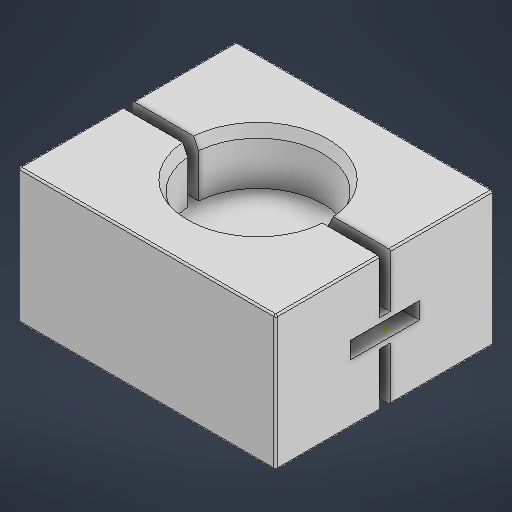
# Autodesk Inventor part: Base_Casing_A0645_v2
Saved by Autodesk Inventor 2026.2 (Build 302298010, 298A)
## iProperties
Created: 2025-09-05
Part Number: Base_Casing_A0645_v2
Material: Generic
Document SubType Name: Modeling
Designer: usman
Density: 1 g/cm^3
Appearance: Default
Author: usman
Autodesk Inventor part; units mm, degrees
ref_plane "YZ Plane" through (0, 0, 0) normal (1, 0, 0) x (0, 1, 0)
ref_plane "XZ Plane" through (0, 0, 0) normal (0, 1, 0) x (-1, 0, 0)
ref_plane "XY Plane" through (0, 0, 0) normal (0, 0, 1) x (1, 0, 0)
sketch "Sketch1" plane through (0, 0, 0) normal (1, 0, 0) x (0, 1, 0)
  line L0 (-39.75, 64.55) -> (39.75, 64.55)
  line L1 (39.75, 64.55) -> (39.75, -64.55)
  line L2 (39.75, -64.55) -> (-39.75, -64.55)
  line L3 (-39.75, -64.55) -> (-39.75, 64.55)
  line L4 (-39.75, 64.55) -> (39.75, -64.55) construction
  line L5 (39.75, 64.55) -> (-39.75, -64.55) construction
  point P0 (0, 0)
  dimension "d0" = 79.5
  dimension "d42" = 129.1
  constraints: 12 end point, 2 midpoint, 2 parallel, 1 horizontal, 1 perpendicular
  measures "d0" distance of L1.end L2.end
  measures "d42" distance of L2.end L0.start
extrude "Extrusion1" add sketch "Sketch1" along normal blind 152.4
sketch "Sketch2" plane through (152.4, 0, 0) normal (1, 0, 0) x (0, 0, -1)
  line L0 (-20.5, -5) -> (20.5, -5)
  line L1 (20.5, -5) -> (20.5, 5)
  line L2 (20.5, 5) -> (-20.5, 5)
  line L3 (-20.5, 5) -> (-20.5, -5)
  line L4 (-20.5, -5) -> (20.5, 5) construction
  line L5 (20.5, -5) -> (-20.5, 5) construction
  point P0 (0, 0)
  dimension "d4" = 10
  dimension "d5" = 41
  constraints: 12 end point, 2 midpoint, 2 parallel, 1 horizontal, 1 perpendicular
  measures "d4" distance of L0.end L1.end
  measures "d5" distance of L1.end L2.end
extrude "Extrusion2" cut sketch "Sketch2" against normal through all
sketch "Sketch3" plane through (152.4, 0, 0) normal (1, 0, 0) x (0, 0, -1)
  point P0 (0, 0)
sketch "Sketch4" plane through (0, 39.75, 64.55) normal (0, 1, 0) x (1, 0, 0)
  line L0 (115.0902, 28.6551) -> (39.7066, 100.4449) construction
  line L1 (39.7066, 28.6551) -> (115.0902, 100.4449) construction
  line L2 (0, 129.1) -> (0, 0) projected
  line L3 (0, 129.1) -> (152.4, 129.1) projected
  circle A0 centre (77.3984, 64.55) radius 38.5
  line L4 (152.4, 129.1) -> (152.4, 0) projected
  point P0 (0, 64.55)
  dimension "d23" = 77
  dimension "d24" = 129.1
  dimension "d25" = 64.55
  dimension "d43" = 77.3984
  dimension "d44" = 75.0016
  constraints: 4 end point, 2 midpoint, 1 centre point, 1 coincident
  measures "d23" diameter of A0
  measures "d24" distance of L2.start L2.end
  measures "d25" vertical distance of point (77.398, 64.55) L2.end
  measures "d43" distance from line of L2 point (77.398, 64.55)
  measures "d44" distance from line of L4 point (77.398, 64.55)
extrude "Extrusion3" cut sketch "Sketch4" against normal blind 31.7
mirror "Mirror1" about plane through (0, 0, 0) normal (0, 1, 0) of "Extrusion3"
sketch "Sketch5" plane through (0, 0, 0) normal (-1, 0, 0) x (0, 0, 1)
  line L0 (-64.55, 39.75) -> (64.55, 39.75) projected
  line L1 (-3.25, 8.05) -> (3.25, 8.05)
  line L2 (3.25, 8.05) -> (3.25, 39.75)
  line L3 (3.25, 39.75) -> (-3.25, 39.75)
  line L4 (-3.25, 39.75) -> (-3.25, 8.05)
  line L5 (-3.25, 8.05) -> (3.25, 39.75) construction
  line L6 (3.25, 8.05) -> (-3.25, 39.75) construction
  point P0 (0, 0)
  point P1 (0, 23.9)
  point P2 (-3.25, 39.75)
  dimension "d12" = 3.25
  dimension "d13" = 31.7
  constraints: 12 end point, 2 midpoint, 2 parallel, 1 horizontal, 1 perpendicular, 1 point on line
  measures "d12" distance from line of point (0, 23.9) L2
  measures "d13" distance of L1.end L2.end
extrude "Extrusion4" cut sketch "Sketch5" against normal through all
mirror "Mirror2" about plane through (0, 0, 0) normal (0, 1, 0) of "Extrusion4"
sketch "Sketch6" plane through (0, 0, 0) normal (-1, 0, 0) x (0, 0, 1)
  line L0 (-53.6471, 38.1768) -> (-14.1529, 38.1768) construction
  line L1 (-14.1529, 38.1768) -> (-14.1529, 7.4202) construction
  line L2 (-14.1529, 7.4202) -> (-53.6471, 7.4202) construction
  line L3 (-53.6471, 7.4202) -> (-53.6471, 38.1768) construction
  line L4 (-64.55, 39.75) -> (-3.25, 39.75) projected
  line L5 (-43.049, 25.8134) -> (-43.049, 31.9094)
  line L6 (-43.049, 31.9094) -> (-42.0942, 31.9094)
  spline S0 degree 2 poles (-42.0942, 31.9094) (-41.2599, 31.9094) (-40.873, 31.8039) knots 0 0 0 1 1 1
  spline S1 degree 2 poles (-40.873, 31.8039) (-40.3302, 31.6581) (-39.6819, 30.8691) (-39.6819, 30.3364) knots 0 0 0 1 2 2 2
  spline S2 degree 2 poles (-39.6819, 30.3364) (-39.6819, 29.9846) (-39.9734, 29.4167) (-40.3051, 29.1705) knots 0 0 0 1 2 2 2
  spline S3 degree 2 poles (-40.3051, 29.1705) (-39.7472, 28.9091) (-39.2346, 28.1252) (-39.2346, 27.5924) knots 0 0 0 1 2 2 2
  spline S4 degree 2 poles (-39.2346, 27.5924) (-39.2346, 27.0748) (-39.7673, 26.2305) (-40.6016, 25.8134) (-41.3403, 25.8134) knots 0 0 0 1 2 3 3 3
  line L7 (-41.3403, 25.8134) -> (-43.049, 25.8134)
  line L8 (-41.8881, 28.482) -> (-41.8881, 26.919)
  line L9 (-41.8881, 26.919) -> (-41.5966, 26.919)
  spline S5 degree 2 poles (-41.5966, 26.919) (-40.878, 26.919) (-40.3754, 27.2859) (-40.3754, 27.6327) knots 0 0 0 1 2 2 2
  spline S6 degree 2 poles (-40.3754, 27.6327) (-40.3754, 28.0246) (-40.9634, 28.482) (-41.6469, 28.482) knots 0 0 0 1 2 2 2
  line L10 (-41.6469, 28.482) -> (-41.8881, 28.482)
  line L11 (-41.8881, 30.8038) -> (-41.8881, 29.5172)
  line L12 (-41.8881, 29.5172) -> (-41.6368, 29.5172)
  spline S7 degree 2 poles (-41.6368, 29.5172) (-41.2147, 29.5172) (-40.8026, 29.8741) (-40.8026, 30.1806) knots 0 0 0 1 2 2 2
  spline S8 degree 2 poles (-40.8026, 30.1806) (-40.8026, 30.4671) (-41.1896, 30.8038) (-41.5916, 30.8038) knots 0 0 0 1 2 2 2
  line L13 (-41.5916, 30.8038) -> (-41.8881, 30.8038)
  line L14 (-34.9227, 30.3213) -> (-33.792, 30.3213)
  line L15 (-33.792, 30.3213) -> (-33.792, 25.8134)
  line L16 (-33.792, 25.8134) -> (-34.9227, 25.8134)
  line L17 (-34.9227, 25.8134) -> (-34.9227, 26.2908)
  spline S9 degree 2 poles (-34.9227, 26.2908) (-35.2544, 25.9742) (-35.9178, 25.6978) (-36.3098, 25.6978) knots 0 0 0 1 2 2 2
  spline S10 degree 2 poles (-36.3098, 25.6978) (-37.1792, 25.6978) (-38.4557, 27.0547) (-38.4557, 28.0598) knots 0 0 0 1 2 2 2
  spline S11 degree 2 poles (-38.4557, 28.0598) (-38.4557, 29.1051) (-37.2244, 30.4369) (-36.3399, 30.4369) knots 0 0 0 1 2 2 2
  spline S12 degree 2 poles (-36.3399, 30.4369) (-35.9379, 30.4369) (-35.2242, 30.1304) (-34.9227, 29.8238) knots 0 0 0 1 2 2 2
  line L18 (-34.9227, 29.8238) -> (-34.9227, 30.3213)
  spline S13 degree 2 poles (-36.1138, 29.3916) (-36.6364, 29.3916) (-37.3299, 28.6528) (-37.3299, 28.0699) knots 0 0 0 1 2 2 2
  spline S14 degree 2 poles (-37.3299, 28.0699) (-37.3299, 27.4869) (-36.6213, 26.7331) (-36.1087, 26.7331) knots 0 0 0 1 2 2 2
  spline S15 degree 2 poles (-36.1087, 26.7331) (-35.576, 26.7331) (-34.8724, 27.4769) (-34.8724, 28.0749) knots 0 0 0 1 2 2 2
  spline S16 degree 2 poles (-34.8724, 28.0749) (-34.8724, 28.6629) (-35.576, 29.3916) (-36.1138, 29.3916) knots 0 0 0 1 2 2 2
  line L19 (-29.8921, 29.6881) -> (-30.5907, 28.9896)
  spline S17 degree 2 poles (-30.5907, 28.9896) (-31.0128, 29.4117) (-31.3596, 29.4117) knots 0 0 0 1 1 1
  spline S18 degree 2 poles (-31.3596, 29.4117) (-31.5506, 29.4117) (-31.7667, 29.2509) (-31.7667, 29.1303) knots 0 0 0 1 2 2 2
  spline S19 degree 2 poles (-31.7667, 29.1303) (-31.7667, 29.0398) (-31.631, 28.884) (-31.3596, 28.7534) knots 0 0 0 1 2 2 2
  line L20 (-31.3596, 28.7534) -> (-30.9475, 28.5473)
  spline S20 degree 2 poles (-30.9475, 28.5473) (-30.2942, 28.2257) (-29.8067, 27.5522) (-29.8067, 27.0999) knots 0 0 0 1 2 2 2
  spline S21 degree 2 poles (-29.8067, 27.0999) (-29.8067, 26.5019) (-30.6862, 25.6978) (-31.4299, 25.6978) knots 0 0 0 1 2 2 2
  spline S22 degree 2 poles (-31.4299, 25.6978) (-32.4149, 25.6978) (-33.0029, 26.4667) knots 0 0 0 1 1 1
  line L21 (-33.0029, 26.4667) -> (-32.3094, 27.2256)
  spline S23 degree 2 poles (-32.3094, 27.2256) (-32.1084, 26.9944) (-31.5757, 26.708) (-31.3696, 26.708) knots 0 0 0 1 2 2 2
  spline S24 degree 2 poles (-31.3696, 26.708) (-31.1435, 26.708) (-30.8721, 26.924) (-30.8721, 27.0648) knots 0 0 0 1 2 2 2
  spline S25 degree 2 poles (-30.8721, 27.0648) (-30.8721, 27.3261) (-31.3646, 27.5723) knots 0 0 0 1 1 1
  line L22 (-31.3646, 27.5723) -> (-31.7465, 27.7633)
  spline S26 degree 2 poles (-31.7465, 27.7633) (-32.8371, 28.3161) (-32.8371, 29.1453) knots 0 0 0 1 1 1
  spline S27 degree 2 poles (-32.8371, 29.1453) (-32.8371, 29.6781) (-32.0129, 30.4369) (-31.3747, 30.4369) knots 0 0 0 1 2 2 2
  spline S28 degree 2 poles (-31.3747, 30.4369) (-30.9324, 30.4369) (-30.1585, 30.0499) (-29.8921, 29.6881) knots 0 0 0 1 2 2 2
  line L23 (-24.3992, 27.7432) -> (-28.0276, 27.7432)
  spline S29 degree 2 poles (-28.0276, 27.7432) (-27.9472, 27.2608) (-27.2638, 26.6929) (-26.7361, 26.6929) knots 0 0 0 1 2 2 2
  spline S30 degree 2 poles (-26.7361, 26.6929) (-26.1028, 26.6929) (-25.6455, 27.1351) knots 0 0 0 1 1 1
  line L24 (-25.6455, 27.1351) -> (-24.6957, 26.6878)
  spline S31 degree 2 poles (-24.6957, 26.6878) (-25.0525, 26.1853) (-26.0476, 25.6978) (-26.731, 25.6978) knots 0 0 0 1 2 2 2
  spline S32 degree 2 poles (-26.731, 25.6978) (-27.7914, 25.6978) (-29.1232, 27.0346) (-29.1232, 28.0447) knots 0 0 0 1 2 2 2
  spline S33 degree 2 poles (-29.1232, 28.0447) (-29.1232, 29.075) (-27.7914, 30.4369) (-26.7914, 30.4369) knots 0 0 0 1 2 2 2
  spline S34 degree 2 poles (-26.7914, 30.4369) (-25.7259, 30.4369) (-24.3942, 29.075) (-24.3942, 27.9593) knots 0 0 0 1 2 2 2
  line L25 (-24.3942, 27.9593) -> (-24.3992, 27.7432)
  spline S35 degree 2 poles (-25.5299, 28.6327) (-25.6405, 29.0097) (-26.2988, 29.477) (-26.7361, 29.477) knots 0 0 0 1 2 2 2
  spline S36 degree 2 poles (-26.7361, 29.477) (-27.2085, 29.477) (-27.5653, 29.2157) knots 0 0 0 1 1 1
  spline S37 degree 2 poles (-27.5653, 29.2157) (-27.7864, 29.0499) (-27.9774, 28.6327) knots 0 0 0 1 1 1
  line L26 (-27.9774, 28.6327) -> (-25.5299, 28.6327)
  line L27 (-48.5721, 21.5476) -> (-47.4464, 21.5476)
  line L28 (-47.4464, 21.5476) -> (-46.0292, 17.296)
  line L29 (-46.0292, 17.296) -> (-44.6019, 21.5476)
  line L30 (-44.6019, 21.5476) -> (-43.4762, 21.5476)
  line L31 (-43.4762, 21.5476) -> (-42.456, 15.4516)
  line L32 (-42.456, 15.4516) -> (-43.5767, 15.4516)
  line L33 (-43.5767, 15.4516) -> (-44.225, 19.3012)
  line L34 (-44.225, 19.3012) -> (-45.5216, 15.4516)
  line L35 (-45.5216, 15.4516) -> (-46.5468, 15.4516)
  line L36 (-46.5468, 15.4516) -> (-47.8283, 19.3012)
  line L37 (-47.8283, 19.3012) -> (-48.4967, 15.4516)
  line L38 (-48.4967, 15.4516) -> (-49.6275, 15.4516)
  line L39 (-49.6275, 15.4516) -> (-48.5721, 21.5476)
  line L40 (-38.32, 19.9595) -> (-37.1892, 19.9595)
  line L41 (-37.1892, 19.9595) -> (-37.1892, 15.4516)
  line L42 (-37.1892, 15.4516) -> (-38.32, 15.4516)
  line L43 (-38.32, 15.4516) -> (-38.32, 15.929)
  spline S38 degree 2 poles (-38.32, 15.929) (-38.6517, 15.6124) (-39.315, 15.336) (-39.707, 15.336) knots 0 0 0 1 2 2 2
  spline S39 degree 2 poles (-39.707, 15.336) (-40.5765, 15.336) (-41.8529, 16.6929) (-41.8529, 17.698) knots 0 0 0 1 2 2 2
  spline S40 degree 2 poles (-41.8529, 17.698) (-41.8529, 18.7433) (-40.6217, 20.0751) (-39.7372, 20.0751) knots 0 0 0 1 2 2 2
  spline S41 degree 2 poles (-39.7372, 20.0751) (-39.3351, 20.0751) (-38.6215, 19.7685) (-38.32, 19.462) knots 0 0 0 1 2 2 2
  line L44 (-38.32, 19.462) -> (-38.32, 19.9595)
  spline S42 degree 2 poles (-39.511, 19.0298) (-40.0337, 19.0298) (-40.7272, 18.291) (-40.7272, 17.7081) knots 0 0 0 1 2 2 2
  spline S43 degree 2 poles (-40.7272, 17.7081) (-40.7272, 17.1251) (-40.0186, 16.3713) (-39.506, 16.3713) knots 0 0 0 1 2 2 2
  spline S44 degree 2 poles (-39.506, 16.3713) (-38.9733, 16.3713) (-38.2697, 17.115) (-38.2697, 17.7131) knots 0 0 0 1 2 2 2
  spline S45 degree 2 poles (-38.2697, 17.7131) (-38.2697, 18.3011) (-38.9733, 19.0298) (-39.511, 19.0298) knots 0 0 0 1 2 2 2
  line L45 (-32.7165, 19.9595) -> (-31.5857, 19.9595)
  line L46 (-31.5857, 19.9595) -> (-31.5857, 16.0999)
  spline S46 degree 2 poles (-31.5857, 16.0999) (-31.5857, 14.9541) (-32.0481, 14.4163) knots 0 0 0 1 1 1
  spline S47 degree 2 poles (-32.0481, 14.4163) (-32.6612, 13.6876) (-33.9075, 13.6876) knots 0 0 0 1 1 1
  spline S48 degree 2 poles (-33.9075, 13.6876) (-34.5709, 13.6876) (-35.4705, 14.0193) (-36.0937, 14.6626) (-36.2444, 15.1199) knots 0 0 0 1 2 3 3 3
  line L47 (-36.2444, 15.1199) -> (-34.9981, 15.1199)
  spline S49 degree 2 poles (-34.9981, 15.1199) (-34.8322, 14.9289) (-34.3096, 14.738) (-33.9528, 14.738) knots 0 0 0 1 2 2 2
  spline S50 degree 2 poles (-33.9528, 14.738) (-33.5005, 14.738) (-32.9426, 15.0194) (-32.7165, 15.4667) (-32.7165, 16.0145) knots 0 0 0 1 2 3 3 3
  spline S51 degree 2 poles (-32.7165, 16.0145) (-33.013, 15.7129) (-33.6663, 15.4516) (-34.0834, 15.4516) knots 0 0 0 1 2 2 2
  spline S52 degree 2 poles (-34.0834, 15.4516) (-34.988, 15.4516) (-36.2394, 16.7633) (-36.2394, 17.7633) knots 0 0 0 1 2 2 2
  spline S53 degree 2 poles (-36.2394, 17.7633) (-36.2394, 18.8388) (-35.576, 19.4871) knots 0 0 0 1 1 1
  spline S54 degree 2 poles (-35.576, 19.4871) (-34.978, 20.0751) (-34.1437, 20.0751) knots 0 0 0 1 1 1
  spline S55 degree 2 poles (-34.1437, 20.0751) (-33.7568, 20.0751) (-33.0632, 19.7886) (-32.7165, 19.462) knots 0 0 0 1 2 2 2
  line L48 (-32.7165, 19.462) -> (-32.7165, 19.9595)
  spline S56 degree 2 poles (-33.8824, 19.0197) (-34.4201, 19.0197) (-35.1137, 18.3011) (-35.1137, 17.7583) knots 0 0 0 1 2 2 2
  spline S57 degree 2 poles (-35.1137, 17.7583) (-35.1137, 17.1955) (-34.4, 16.4768) (-33.8623, 16.4768) knots 0 0 0 1 2 2 2
  spline S58 degree 2 poles (-33.8623, 16.4768) (-33.3396, 16.4768) (-32.6562, 17.1804) (-32.6562, 17.7533) knots 0 0 0 1 2 2 2
  spline S59 degree 2 poles (-32.6562, 17.7533) (-32.6562, 18.3162) (-33.3447, 19.0197) (-33.8824, 19.0197) knots 0 0 0 1 2 2 2
  line L49 (-30.4399, 19.9595) -> (-29.3092, 19.9595)
  line L50 (-29.3092, 19.9595) -> (-29.3092, 19.4972)
  spline S60 degree 2 poles (-29.3092, 19.4972) (-28.9222, 19.8238) (-28.299, 20.0751) (-27.9724, 20.0751) knots 0 0 0 1 2 2 2
  spline S61 degree 2 poles (-27.9724, 20.0751) (-27.2989, 20.0751) (-26.8316, 19.6077) knots 0 0 0 1 1 1
  spline S62 degree 2 poles (-26.8316, 19.6077) (-26.4396, 19.2107) (-26.4396, 18.4317) knots 0 0 0 1 1 1
  line L51 (-26.4396, 18.4317) -> (-26.4396, 15.4516)
  line L52 (-26.4396, 15.4516) -> (-27.5603, 15.4516)
  line L53 (-27.5603, 15.4516) -> (-27.5603, 17.4266)
  spline S63 degree 2 poles (-27.5603, 17.4266) (-27.5603, 18.2307) (-27.706, 18.7634) (-28.0628, 19.0398) (-28.3292, 19.0398) knots 0 0 0 1 2 3 3 3
  spline S64 degree 2 poles (-28.3292, 19.0398) (-28.6709, 19.0398) (-29.1634, 18.5825) (-29.2589, 18.1754) knots 0 0 0 1 2 2 2
  spline S65 degree 2 poles (-29.2589, 18.1754) (-29.3092, 17.9644) (-29.3092, 17.2608) knots 0 0 0 1 1 1
  line L54 (-29.3092, 17.2608) -> (-29.3092, 15.4516)
  line L55 (-29.3092, 15.4516) -> (-30.4399, 15.4516)
  line L56 (-30.4399, 15.4516) -> (-30.4399, 19.9595)
  line L57 (-20.831, 17.3814) -> (-24.4595, 17.3814)
  spline S66 degree 2 poles (-24.4595, 17.3814) (-24.3791, 16.8989) (-23.6956, 16.3311) (-23.1679, 16.3311) knots 0 0 0 1 2 2 2
  spline S67 degree 2 poles (-23.1679, 16.3311) (-22.5347, 16.3311) (-22.0774, 16.7733) knots 0 0 0 1 1 1
  line L58 (-22.0774, 16.7733) -> (-21.1275, 16.326)
  spline S68 degree 2 poles (-21.1275, 16.326) (-21.4844, 15.8235) (-22.4794, 15.336) (-23.1629, 15.336) knots 0 0 0 1 2 2 2
  spline S69 degree 2 poles (-23.1629, 15.336) (-24.2233, 15.336) (-25.5551, 16.6728) (-25.5551, 17.6829) knots 0 0 0 1 2 2 2
  spline S70 degree 2 poles (-25.5551, 17.6829) (-25.5551, 18.7132) (-24.2233, 20.0751) (-23.2232, 20.0751) knots 0 0 0 1 2 2 2
  spline S71 degree 2 poles (-23.2232, 20.0751) (-22.1578, 20.0751) (-20.826, 18.7132) (-20.826, 17.5975) knots 0 0 0 1 2 2 2
  line L59 (-20.826, 17.5975) -> (-20.831, 17.3814)
  spline S72 degree 2 poles (-21.9618, 18.2709) (-22.0724, 18.6478) (-22.7307, 19.1152) (-23.1679, 19.1152) knots 0 0 0 1 2 2 2
  spline S73 degree 2 poles (-23.1679, 19.1152) (-23.6403, 19.1152) (-23.9971, 18.8539) knots 0 0 0 1 1 1
  spline S74 degree 2 poles (-23.9971, 18.8539) (-24.2183, 18.688) (-24.4092, 18.2709) knots 0 0 0 1 1 1
  line L60 (-24.4092, 18.2709) -> (-21.9618, 18.2709)
  line L61 (-19.7757, 21.623) -> (-18.6449, 21.623)
  line L62 (-18.6449, 21.623) -> (-18.6449, 19.9595)
  line L63 (-18.6449, 19.9595) -> (-17.9715, 19.9595)
  line L64 (-17.9715, 19.9595) -> (-17.9715, 18.9846)
  line L65 (-17.9715, 18.9846) -> (-18.6449, 18.9846)
  line L66 (-18.6449, 18.9846) -> (-18.6449, 15.4516)
  line L67 (-18.6449, 15.4516) -> (-19.7757, 15.4516)
  line L68 (-19.7757, 15.4516) -> (-19.7757, 18.9846)
  line L69 (-19.7757, 18.9846) -> (-20.3536, 18.9846)
  line L70 (-20.3536, 18.9846) -> (-20.3536, 19.9595)
  line L71 (-20.3536, 19.9595) -> (-19.7757, 19.9595)
  line L72 (-19.7757, 19.9595) -> (-19.7757, 21.623)
  point P0 (0, 0)
  point P1 (-33.9, 39.75)
  point P2 (-33.9, 38.1768)
  dimension "d0" = 79.5
  dimension "d42" = 129.1
  dimension "d26" = 0
  constraints: 2 midpoint, 2 other
  measures "d26" horizontal distance of point (-33.9, 39.75) point (-33.9, 38.177)
sketch "Sketch7" plane through (0, 0, 0) normal (-1, 0, 0) x (0, 0, 1)
  line L0 (15.2014, 37.9215) -> (52.5986, 37.9215) construction
  line L1 (52.5986, 37.9215) -> (52.5986, 6.8154) construction
  line L2 (52.5986, 6.8154) -> (15.2014, 6.8154) construction
  line L3 (15.2014, 6.8154) -> (15.2014, 37.9215) construction
  line L4 (-52.3897, -8.5629) -> (-15.4103, -8.5629) construction
  line L5 (-15.4103, -8.5629) -> (-15.4103, -37.9215) construction
  line L6 (-15.4103, -37.9215) -> (-52.3897, -37.9215) construction
  line L7 (-52.3897, -37.9215) -> (-52.3897, -8.5629) construction
  line L8 (3.25, 39.75) -> (64.55, 39.75) projected
  line L9 (-3.25, -39.75) -> (-64.55, -39.75) projected
  line L10 (25.8516, 25.0873) -> (25.0425, 24.3133)
  spline S0 degree 2 poles (25.0425, 24.3133) (24.2132, 25.1878) (23.178, 25.1878) knots 0 0 0 1 1 1
  spline S1 degree 2 poles (23.178, 25.1878) (22.3035, 25.1878) (21.1074, 23.9967) (21.1074, 23.1223) knots 0 0 0 1 2 2 2
  spline S2 degree 2 poles (21.1074, 23.1223) (21.1074, 22.5142) (21.6351, 21.5694) (22.6051, 21.0316) (23.1981, 21.0316) knots 0 0 0 1 2 3 3 3
  spline S3 degree 2 poles (23.1981, 21.0316) (23.7006, 21.0316) (24.5399, 21.4085) (25.0425, 21.9061) knots 0 0 0 1 2 2 2
  line L11 (25.0425, 21.9061) -> (25.8264, 21.0869)
  spline S4 degree 2 poles (25.8264, 21.0869) (25.153, 20.4235) (23.9519, 19.916) (23.178, 19.916) knots 0 0 0 1 2 2 2
  spline S5 degree 2 poles (23.178, 19.916) (21.7557, 19.916) (19.9465, 21.7151) (19.9465, 23.1273) knots 0 0 0 1 2 2 2
  spline S6 degree 2 poles (19.9465, 23.1273) (19.9465, 24.0369) (20.7707, 25.4541) (22.3086, 26.3135) (23.1931, 26.3135) knots 0 0 0 1 2 3 3 3
  spline S7 degree 2 poles (23.1931, 26.3135) (23.9519, 26.3135) (25.344, 25.6752) (25.8516, 25.0873) knots 0 0 0 1 2 2 2
  line L12 (30.073, 24.5746) -> (31.2038, 24.5746)
  line L13 (31.2038, 24.5746) -> (31.2038, 20.0667)
  line L14 (31.2038, 20.0667) -> (30.073, 20.0667)
  line L15 (30.073, 20.0667) -> (30.073, 20.5442)
  spline S8 degree 2 poles (30.073, 20.5442) (29.7414, 20.2275) (29.078, 19.9511) (28.686, 19.9511) knots 0 0 0 1 2 2 2
  spline S9 degree 2 poles (28.686, 19.9511) (27.8166, 19.9511) (26.5401, 21.308) (26.5401, 22.3131) knots 0 0 0 1 2 2 2
  spline S10 degree 2 poles (26.5401, 22.3131) (26.5401, 23.3585) (27.7713, 24.6902) (28.6558, 24.6902) knots 0 0 0 1 2 2 2
  spline S11 degree 2 poles (28.6558, 24.6902) (29.0579, 24.6902) (29.7715, 24.3837) (30.073, 24.0771) knots 0 0 0 1 2 2 2
  line L16 (30.073, 24.0771) -> (30.073, 24.5746)
  spline S12 degree 2 poles (28.882, 23.6449) (28.3593, 23.6449) (27.6658, 22.9062) (27.6658, 22.3232) knots 0 0 0 1 2 2 2
  spline S13 degree 2 poles (27.6658, 22.3232) (27.6658, 21.7402) (28.3744, 20.9864) (28.887, 20.9864) knots 0 0 0 1 2 2 2
  spline S14 degree 2 poles (28.887, 20.9864) (29.4197, 20.9864) (30.1233, 21.7302) (30.1233, 22.3282) knots 0 0 0 1 2 2 2
  spline S15 degree 2 poles (30.1233, 22.3282) (30.1233, 22.9162) (29.4197, 23.6449) (28.882, 23.6449) knots 0 0 0 1 2 2 2
  line L17 (35.1036, 23.9414) -> (34.4051, 23.2429)
  spline S16 degree 2 poles (34.4051, 23.2429) (33.9829, 23.665) (33.6362, 23.665) knots 0 0 0 1 1 1
  spline S17 degree 2 poles (33.6362, 23.665) (33.4452, 23.665) (33.2291, 23.5042) (33.2291, 23.3836) knots 0 0 0 1 2 2 2
  spline S18 degree 2 poles (33.2291, 23.3836) (33.2291, 23.2931) (33.3648, 23.1373) (33.6362, 23.0067) knots 0 0 0 1 2 2 2
  line L18 (33.6362, 23.0067) -> (34.0483, 22.8006)
  spline S19 degree 2 poles (34.0483, 22.8006) (34.7016, 22.479) (35.1891, 21.8056) (35.1891, 21.3533) knots 0 0 0 1 2 2 2
  spline S20 degree 2 poles (35.1891, 21.3533) (35.1891, 20.7552) (34.3096, 19.9511) (33.5658, 19.9511) knots 0 0 0 1 2 2 2
  spline S21 degree 2 poles (33.5658, 19.9511) (32.5808, 19.9511) (31.9928, 20.72) knots 0 0 0 1 1 1
  line L19 (31.9928, 20.72) -> (32.6863, 21.4789)
  spline S22 degree 2 poles (32.6863, 21.4789) (32.8874, 21.2477) (33.4201, 20.9613) (33.6261, 20.9613) knots 0 0 0 1 2 2 2
  spline S23 degree 2 poles (33.6261, 20.9613) (33.8523, 20.9613) (34.1236, 21.1774) (34.1236, 21.3181) knots 0 0 0 1 2 2 2
  spline S24 degree 2 poles (34.1236, 21.3181) (34.1236, 21.5794) (33.6311, 21.8257) knots 0 0 0 1 1 1
  line L20 (33.6311, 21.8257) -> (33.2492, 22.0166)
  spline S25 degree 2 poles (33.2492, 22.0166) (32.1586, 22.5695) (32.1586, 23.3987) knots 0 0 0 1 1 1
  spline S26 degree 2 poles (32.1586, 23.3987) (32.1586, 23.9314) (32.9828, 24.6902) (33.6211, 24.6902) knots 0 0 0 1 2 2 2
  spline S27 degree 2 poles (33.6211, 24.6902) (34.0633, 24.6902) (34.8373, 24.3033) (35.1036, 23.9414) knots 0 0 0 1 2 2 2
  line L21 (35.958, 24.5746) -> (37.0887, 24.5746)
  line L22 (37.0887, 24.5746) -> (37.0887, 20.0667)
  line L23 (37.0887, 20.0667) -> (35.958, 20.0667)
  line L24 (35.958, 20.0667) -> (35.958, 24.5746)
  spline S28 degree 2 poles (36.5208, 26.4341) (36.8173, 26.4341) (37.2445, 26.0019) (37.2445, 25.6953) knots 0 0 0 1 2 2 2
  spline S29 degree 2 poles (37.2445, 25.6953) (37.2445, 25.3938) (36.8224, 24.9666) (36.5309, 24.9666) knots 0 0 0 1 2 2 2
  spline S30 degree 2 poles (36.5309, 24.9666) (36.2293, 24.9666) (35.8022, 25.4039) (35.8022, 25.7104) knots 0 0 0 1 2 2 2
  spline S31 degree 2 poles (35.8022, 25.7104) (35.8022, 26.012) (36.2243, 26.4341) (36.5208, 26.4341) knots 0 0 0 1 2 2 2
  line L25 (38.119, 24.5746) -> (39.2497, 24.5746)
  line L26 (39.2497, 24.5746) -> (39.2497, 24.1123)
  spline S32 degree 2 poles (39.2497, 24.1123) (39.6367, 24.439) (40.2598, 24.6902) (40.5865, 24.6902) knots 0 0 0 1 2 2 2
  spline S33 degree 2 poles (40.5865, 24.6902) (41.2599, 24.6902) (41.7273, 24.2229) knots 0 0 0 1 1 1
  spline S34 degree 2 poles (41.7273, 24.2229) (42.1193, 23.8258) (42.1193, 23.0469) knots 0 0 0 1 1 1
  line L27 (42.1193, 23.0469) -> (42.1193, 20.0667)
  line L28 (42.1193, 20.0667) -> (40.9986, 20.0667)
  line L29 (40.9986, 20.0667) -> (40.9986, 22.0418)
  spline S35 degree 2 poles (40.9986, 22.0418) (40.9986, 22.8459) (40.8529, 23.3786) (40.496, 23.655) (40.2297, 23.655) knots 0 0 0 1 2 3 3 3
  spline S36 degree 2 poles (40.2297, 23.655) (39.888, 23.655) (39.3954, 23.1976) (39.3, 22.7906) knots 0 0 0 1 2 2 2
  spline S37 degree 2 poles (39.3, 22.7906) (39.2497, 22.5795) (39.2497, 21.8759) knots 0 0 0 1 1 1
  line L30 (39.2497, 21.8759) -> (39.2497, 20.0667)
  line L31 (39.2497, 20.0667) -> (38.119, 20.0667)
  line L32 (38.119, 20.0667) -> (38.119, 24.5746)
  line L33 (46.5418, 24.5746) -> (47.6725, 24.5746)
  line L34 (47.6725, 24.5746) -> (47.6725, 20.715)
  spline S38 degree 2 poles (47.6725, 20.715) (47.6725, 19.5692) (47.2102, 19.0315) knots 0 0 0 1 1 1
  spline S39 degree 2 poles (47.2102, 19.0315) (46.5971, 18.3028) (45.3507, 18.3028) knots 0 0 0 1 1 1
  spline S40 degree 2 poles (45.3507, 18.3028) (44.6874, 18.3028) (43.7878, 18.6344) (43.1646, 19.2777) (43.0138, 19.735) knots 0 0 0 1 2 3 3 3
  line L35 (43.0138, 19.735) -> (44.2602, 19.735)
  spline S41 degree 2 poles (44.2602, 19.735) (44.426, 19.5441) (44.9487, 19.3531) (45.3055, 19.3531) knots 0 0 0 1 2 2 2
  spline S42 degree 2 poles (45.3055, 19.3531) (45.7578, 19.3531) (46.3156, 19.6345) (46.5418, 20.0818) (46.5418, 20.6296) knots 0 0 0 1 2 3 3 3
  spline S43 degree 2 poles (46.5418, 20.6296) (46.2453, 20.3281) (45.592, 20.0667) (45.1748, 20.0667) knots 0 0 0 1 2 2 2
  spline S44 degree 2 poles (45.1748, 20.0667) (44.2702, 20.0667) (43.0189, 21.3784) (43.0189, 22.3785) knots 0 0 0 1 2 2 2
  spline S45 degree 2 poles (43.0189, 22.3785) (43.0189, 23.4539) (43.6822, 24.1022) knots 0 0 0 1 1 1
  spline S46 degree 2 poles (43.6822, 24.1022) (44.2803, 24.6902) (45.1145, 24.6902) knots 0 0 0 1 1 1
  spline S47 degree 2 poles (45.1145, 24.6902) (45.5015, 24.6902) (46.195, 24.4038) (46.5418, 24.0771) knots 0 0 0 1 2 2 2
  line L36 (46.5418, 24.0771) -> (46.5418, 24.5746)
  spline S48 degree 2 poles (45.3759, 23.6349) (44.8381, 23.6349) (44.1446, 22.9162) (44.1446, 22.3735) knots 0 0 0 1 2 2 2
  spline S49 degree 2 poles (44.1446, 22.3735) (44.1446, 21.8106) (44.8582, 21.0919) (45.396, 21.0919) knots 0 0 0 1 2 2 2
  spline S50 degree 2 poles (45.396, 21.0919) (45.9186, 21.0919) (46.6021, 21.7955) (46.6021, 22.3684) knots 0 0 0 1 2 2 2
  spline S51 degree 2 poles (46.6021, 22.3684) (46.6021, 22.9313) (45.9136, 23.6349) (45.3759, 23.6349) knots 0 0 0 1 2 2 2
  line L37 (-51.1251, -20.1942) -> (-49.9441, -20.1942)
  line L38 (-49.9441, -20.1942) -> (-47.6022, -26.2902)
  line L39 (-47.6022, -26.2902) -> (-48.8083, -26.2902)
  line L40 (-48.8083, -26.2902) -> (-49.2857, -25.0338)
  line L41 (-49.2857, -25.0338) -> (-51.7734, -25.0338)
  line L42 (-51.7734, -25.0338) -> (-52.2659, -26.2902)
  line L43 (-52.2659, -26.2902) -> (-53.472, -26.2902)
  line L44 (-53.472, -26.2902) -> (-51.1251, -20.1942)
  line L45 (-50.5271, -21.8124) -> (-51.3462, -23.9031)
  line L46 (-51.3462, -23.9031) -> (-49.7179, -23.9031)
  line L47 (-49.7179, -23.9031) -> (-50.5271, -21.8124)
  spline S52 degree 2 poles (-45.0442, -20.0434) (-44.3758, -20.0434) (-43.4109, -20.6968) (-42.8832, -22.0436) (-42.8832, -23.2447) knots 0 0 0 1 2 3 3 3
  spline S53 degree 2 poles (-42.8832, -23.2447) (-42.8832, -24.4559) (-43.4159, -25.8077) (-44.3205, -26.441) (-45.009, -26.441) knots 0 0 0 1 2 3 3 3
  spline S54 degree 2 poles (-45.009, -26.441) (-45.6975, -26.441) (-46.6322, -25.8027) (-47.165, -24.5011) (-47.165, -23.3) knots 0 0 0 1 2 3 3 3
  spline S55 degree 2 poles (-47.165, -23.3) (-47.165, -21.6265) (-46.6473, -20.8726) knots 0 0 0 1 1 1
  spline S56 degree 2 poles (-46.6473, -20.8726) (-46.0694, -20.0434) (-45.0442, -20.0434) knots 0 0 0 1 1 1
  spline S57 degree 2 poles (-45.014, -21.144) (-45.3105, -21.144) (-45.7628, -21.5209) (-46.0041, -22.4406) (-46.0041, -23.3251) knots 0 0 0 1 2 3 3 3
  spline S58 degree 2 poles (-46.0041, -23.3251) (-46.0041, -24.481) (-45.4563, -25.3655) (-45.014, -25.3655) knots 0 0 0 1 2 2 2
  spline S59 degree 2 poles (-45.014, -25.3655) (-44.5919, -25.3655) (-44.3456, -24.9484) knots 0 0 0 1 1 1
  spline S60 degree 2 poles (-44.3456, -24.9484) (-44.0441, -24.4408) (-44.0441, -23.2548) knots 0 0 0 1 1 1
  spline S61 degree 2 poles (-44.0441, -23.2548) (-44.0441, -22.0537) (-44.5868, -21.144) (-45.014, -21.144) knots 0 0 0 1 2 2 2
  line L48 (-40.1895, -20.0434) -> (-39.2045, -20.5359)
  line L49 (-39.2045, -20.5359) -> (-40.2649, -22.6115)
  spline S62 degree 2 poles (-40.2649, -22.6115) (-39.4909, -22.6115) (-38.4054, -23.7221) (-38.4054, -24.5413) knots 0 0 0 1 2 2 2
  spline S63 degree 2 poles (-38.4054, -24.5413) (-38.4054, -25.3353) (-39.5211, -26.441) (-40.3051, -26.441) knots 0 0 0 1 2 2 2
  spline S64 degree 2 poles (-40.3051, -26.441) (-41.1343, -26.441) (-42.2299, -25.2951) (-42.2299, -24.5564) knots 0 0 0 1 2 2 2
  spline S65 degree 2 poles (-42.2299, -24.5564) (-42.2299, -24.2749) (-42.059, -23.7071) (-41.7524, -23.114) knots 0 0 0 1 2 2 2
  line L50 (-41.7524, -23.114) -> (-40.1895, -20.0434)
  spline S66 degree 2 poles (-40.3302, -23.7121) (-40.6569, -23.7121) (-41.0941, -24.1795) (-41.0941, -24.5262) knots 0 0 0 1 2 2 2
  spline S67 degree 2 poles (-41.0941, -24.5262) (-41.0941, -24.878) (-40.6368, -25.3554) (-40.3302, -25.3554) knots 0 0 0 1 2 2 2
  spline S68 degree 2 poles (-40.3302, -25.3554) (-40.0035, -25.3554) (-39.5412, -24.8881) (-39.5412, -24.5262) knots 0 0 0 1 2 2 2
  spline S69 degree 2 poles (-39.5412, -24.5262) (-39.5412, -24.1795) (-39.9935, -23.7121) (-40.3302, -23.7121) knots 0 0 0 1 2 2 2
  line L51 (-35.0735, -20.0434) -> (-33.9226, -20.0434)
  line L52 (-33.9226, -20.0434) -> (-33.9226, -23.9634)
  line L53 (-33.9226, -23.9634) -> (-33.3799, -23.9634)
  line L54 (-33.3799, -23.9634) -> (-33.3799, -25.0388)
  line L55 (-33.3799, -25.0388) -> (-33.9226, -25.0388)
  line L56 (-33.9226, -25.0388) -> (-33.9226, -26.2902)
  line L57 (-33.9226, -26.2902) -> (-35.0584, -26.2902)
  line L58 (-35.0584, -26.2902) -> (-35.0584, -25.0388)
  line L59 (-35.0584, -25.0388) -> (-37.7169, -25.0388)
  line L60 (-37.7169, -25.0388) -> (-37.7169, -23.9634)
  line L61 (-37.7169, -23.9634) -> (-35.0735, -20.0434)
  line L62 (-35.0584, -23.9634) -> (-35.0584, -21.923)
  line L63 (-35.0584, -21.923) -> (-36.4505, -23.9634)
  line L64 (-36.4505, -23.9634) -> (-35.0584, -23.9634)
  line L65 (-31.7214, -20.1942) -> (-28.8669, -20.1942)
  line L66 (-28.8669, -20.1942) -> (-28.8669, -21.2697)
  line L67 (-28.8669, -21.2697) -> (-30.857, -21.2697)
  line L68 (-30.857, -21.2697) -> (-31.1033, -22.3753)
  spline S70 degree 2 poles (-31.1033, -22.3753) (-30.9977, -22.3451) (-30.8017, -22.315) (-30.7113, -22.315) knots 0 0 0 1 2 2 2
  spline S71 degree 2 poles (-30.7113, -22.315) (-29.8821, -22.315) (-28.7815, -23.4457) (-28.7815, -24.3302) knots 0 0 0 1 2 2 2
  spline S72 degree 2 poles (-28.7815, -24.3302) (-28.7815, -25.2198) (-29.9977, -26.441) (-30.8671, -26.441) knots 0 0 0 1 2 2 2
  spline S73 degree 2 poles (-30.8671, -26.441) (-31.646, -26.441) (-32.7617, -25.5565) (-32.9376, -24.7876) knots 0 0 0 1 2 2 2
  line L69 (-32.9376, -24.7876) -> (-31.7214, -24.7876)
  spline S74 degree 2 poles (-31.7214, -24.7876) (-31.5807, -25.074) (-31.1184, -25.3655) (-30.8419, -25.3655) knots 0 0 0 1 2 2 2
  spline S75 degree 2 poles (-30.8419, -25.3655) (-30.455, -25.3655) (-29.9172, -24.8127) (-29.9172, -24.3755) knots 0 0 0 1 2 2 2
  spline S76 degree 2 poles (-29.9172, -24.3755) (-29.9172, -23.9533) (-30.4198, -23.4106) (-30.7766, -23.4106) knots 0 0 0 1 2 2 2
  spline S77 degree 2 poles (-30.7766, -23.4106) (-30.9676, -23.4106) (-31.3345, -23.6015) (-31.5103, -23.7925) knots 0 0 0 1 2 2 2
  line L70 (-31.5103, -23.7925) -> (-32.4602, -23.5814)
  line L71 (-32.4602, -23.5814) -> (-31.7214, -20.1942)
  spline S78 degree 2 poles (-26.0275, -20.0434) (-25.3591, -20.0434) (-24.3942, -20.6968) (-23.8665, -22.0436) (-23.8665, -23.2447) knots 0 0 0 1 2 3 3 3
  spline S79 degree 2 poles (-23.8665, -23.2447) (-23.8665, -24.4559) (-24.3992, -25.8077) (-25.3038, -26.441) (-25.9923, -26.441) knots 0 0 0 1 2 3 3 3
  spline S80 degree 2 poles (-25.9923, -26.441) (-26.6808, -26.441) (-27.6155, -25.8027) (-28.1482, -24.5011) (-28.1482, -23.3) knots 0 0 0 1 2 3 3 3
  spline S81 degree 2 poles (-28.1482, -23.3) (-28.1482, -21.6265) (-27.6306, -20.8726) knots 0 0 0 1 1 1
  spline S82 degree 2 poles (-27.6306, -20.8726) (-27.0527, -20.0434) (-26.0275, -20.0434) knots 0 0 0 1 1 1
  spline S83 degree 2 poles (-25.9973, -21.144) (-26.2938, -21.144) (-26.7461, -21.5209) (-26.9873, -22.4406) (-26.9873, -23.3251) knots 0 0 0 1 2 3 3 3
  spline S84 degree 2 poles (-26.9873, -23.3251) (-26.9873, -24.481) (-26.4396, -25.3655) (-25.9973, -25.3655) knots 0 0 0 1 2 2 2
  spline S85 degree 2 poles (-25.9973, -25.3655) (-25.5752, -25.3655) (-25.3289, -24.9484) knots 0 0 0 1 1 1
  spline S86 degree 2 poles (-25.3289, -24.9484) (-25.0274, -24.4408) (-25.0274, -23.2548) knots 0 0 0 1 1 1
  spline S87 degree 2 poles (-25.0274, -23.2548) (-25.0274, -22.0537) (-25.5701, -21.144) (-25.9973, -21.144) knots 0 0 0 1 2 2 2
  spline S88 degree 2 poles (-21.2733, -20.0434) (-20.6049, -20.0434) (-19.64, -20.6968) (-19.1123, -22.0436) (-19.1123, -23.2447) knots 0 0 0 1 2 3 3 3
  spline S89 degree 2 poles (-19.1123, -23.2447) (-19.1123, -24.4559) (-19.645, -25.8077) (-20.5496, -26.441) (-21.2381, -26.441) knots 0 0 0 1 2 3 3 3
  spline S90 degree 2 poles (-21.2381, -26.441) (-21.9266, -26.441) (-22.8614, -25.8027) (-23.3941, -24.5011) (-23.3941, -23.3) knots 0 0 0 1 2 3 3 3
  spline S91 degree 2 poles (-23.3941, -23.3) (-23.3941, -21.6265) (-22.8764, -20.8726) knots 0 0 0 1 1 1
  spline S92 degree 2 poles (-22.8764, -20.8726) (-22.2985, -20.0434) (-21.2733, -20.0434) knots 0 0 0 1 1 1
  spline S93 degree 2 poles (-21.2431, -21.144) (-21.5396, -21.144) (-21.9919, -21.5209) (-22.2332, -22.4406) (-22.2332, -23.3251) knots 0 0 0 1 2 3 3 3
  spline S94 degree 2 poles (-22.2332, -23.3251) (-22.2332, -24.481) (-21.6854, -25.3655) (-21.2431, -25.3655) knots 0 0 0 1 2 2 2
  spline S95 degree 2 poles (-21.2431, -25.3655) (-20.821, -25.3655) (-20.5747, -24.9484) knots 0 0 0 1 1 1
  spline S96 degree 2 poles (-20.5747, -24.9484) (-20.2732, -24.4408) (-20.2732, -23.2548) knots 0 0 0 1 1 1
  spline S97 degree 2 poles (-20.2732, -23.2548) (-20.2732, -22.0537) (-20.816, -21.144) (-21.2431, -21.144) knots 0 0 0 1 2 2 2
  line L72 (-17.479, -20.1942) -> (-15.7452, -20.1942)
  line L73 (-15.7452, -20.1942) -> (-15.7452, -26.2902)
  line L74 (-15.7452, -26.2902) -> (-16.896, -26.2902)
  line L75 (-16.896, -26.2902) -> (-16.896, -21.2847)
  line L76 (-16.896, -21.2847) -> (-18.1524, -21.2847)
  line L77 (-18.1524, -21.2847) -> (-17.479, -20.1942)
  point P0 (0, 0)
  point P1 (33.9, 39.75)
  point P2 (33.9, 37.9215)
  point P3 (-33.9, -39.75)
  point P4 (-33.9, -37.9215)
  dimension "d0" = 79.5
  dimension "d42" = 129.1
  dimension "d27" = 0
  dimension "d28" = 0
  constraints: 4 midpoint, 4 other
  measures "d27" horizontal distance of point (33.9, 39.75) point (33.9, 37.921)
  measures "d28" horizontal distance of point (-33.9, -39.75) point (-33.9, -37.921)
sketch "Sketch8" plane through (0, 0, 0) normal (-1, 0, 0) x (0, 0, 1)
  line L0 (15.5509, -8.5629) -> (52.2491, -8.5629) construction
  line L1 (52.2491, -8.5629) -> (52.2491, -38.6205) construction
  line L2 (52.2491, -38.6205) -> (15.5509, -38.6205) construction
  line L3 (15.5509, -38.6205) -> (15.5509, -8.5629) construction
  line L4 (64.55, -39.75) -> (3.25, -39.75) projected
  line L5 (18.0594, -17.3303) -> (16.9287, -17.3303)
  spline S0 degree 2 poles (16.9287, -17.3303) (16.9739, -16.3453) (18.1248, -15.2145) (19.0244, -15.2145) knots 0 0 0 1 2 2 2
  spline S1 degree 2 poles (19.0244, -15.2145) (19.5772, -15.2145) (20.4315, -15.6819) (20.9391, -16.5664) (20.9391, -17.0187) knots 0 0 0 1 2 3 3 3
  spline S2 degree 2 poles (20.9391, -17.0187) (20.9391, -17.5615) (20.3209, -18.8128) (19.4968, -19.6672) knots 0 0 0 1 2 2 2
  line L6 (19.4968, -19.6672) -> (18.8133, -20.3858)
  line L7 (18.8133, -20.3858) -> (20.9893, -20.3858)
  line L8 (20.9893, -20.3858) -> (20.9893, -21.4613)
  line L9 (20.9893, -21.4613) -> (16.7629, -21.4613)
  line L10 (16.7629, -21.4613) -> (16.7629, -20.9085)
  line L11 (16.7629, -20.9085) -> (18.6525, -18.9837)
  spline S3 degree 2 poles (18.6525, -18.9837) (19.3359, -18.2902) (19.7882, -17.4509) (19.7882, -17.1142) knots 0 0 0 1 2 2 2
  spline S4 degree 2 poles (19.7882, -17.1142) (19.7882, -16.7574) (19.3209, -16.3001) (18.949, -16.3001) knots 0 0 0 1 2 2 2
  spline S5 degree 2 poles (18.949, -16.3001) (18.5771, -16.3001) (18.0745, -16.8529) (18.0594, -17.3303) knots 0 0 0 1 2 2 2
  line L12 (21.8437, -15.3653) -> (25.844, -15.3653)
  line L13 (25.844, -15.3653) -> (25.844, -15.9734)
  line L14 (25.844, -15.9734) -> (23.09, -21.6121)
  line L15 (23.09, -21.6121) -> (22.11, -21.1346)
  line L16 (22.11, -21.1346) -> (24.3967, -16.4559)
  line L17 (24.3967, -16.4559) -> (21.8437, -16.4559)
  line L18 (21.8437, -16.4559) -> (21.8437, -15.3653)
  line L19 (26.7989, -15.2899) -> (27.9296, -15.2899)
  line L20 (27.9296, -15.2899) -> (27.9296, -16.9534)
  line L21 (27.9296, -16.9534) -> (28.6031, -16.9534)
  line L22 (28.6031, -16.9534) -> (28.6031, -17.9283)
  line L23 (28.6031, -17.9283) -> (27.9296, -17.9283)
  line L24 (27.9296, -17.9283) -> (27.9296, -21.4613)
  line L25 (27.9296, -21.4613) -> (26.7989, -21.4613)
  line L26 (26.7989, -21.4613) -> (26.7989, -17.9283)
  line L27 (26.7989, -17.9283) -> (26.2209, -17.9283)
  line L28 (26.2209, -17.9283) -> (26.2209, -16.9534)
  line L29 (26.2209, -16.9534) -> (26.7989, -16.9534)
  line L30 (26.7989, -16.9534) -> (26.7989, -15.2899)
  line L31 (29.2112, -15.2095) -> (30.3319, -15.2095)
  line L32 (30.3319, -15.2095) -> (30.3319, -17.4107)
  spline S6 degree 2 poles (30.3319, -17.4107) (30.6635, -17.1243) (31.337, -16.8378) (31.6787, -16.8378) knots 0 0 0 1 2 2 2
  spline S7 degree 2 poles (31.6787, -16.8378) (32.3521, -16.8378) (32.8145, -17.3001) knots 0 0 0 1 1 1
  spline S8 degree 2 poles (32.8145, -17.3001) (33.2065, -17.7022) (33.2065, -18.4812) knots 0 0 0 1 1 1
  line L33 (33.2065, -18.4812) -> (33.2065, -21.4613)
  line L34 (33.2065, -21.4613) -> (32.0908, -21.4613)
  line L35 (32.0908, -21.4613) -> (32.0908, -19.4863)
  spline S9 degree 2 poles (32.0908, -19.4863) (32.0908, -18.7023) (31.94, -18.1444) (31.5782, -17.8731) (31.3169, -17.8731) knots 0 0 0 1 2 3 3 3
  spline S10 degree 2 poles (31.3169, -17.8731) (30.9701, -17.8731) (30.4776, -18.3304) (30.3821, -18.7224) knots 0 0 0 1 2 2 2
  spline S11 degree 2 poles (30.3821, -18.7224) (30.3319, -18.9234) (30.3319, -19.6521) knots 0 0 0 1 1 1
  line L36 (30.3319, -19.6521) -> (30.3319, -21.4613)
  line L37 (30.3319, -21.4613) -> (29.2112, -21.4613)
  line L38 (29.2112, -21.4613) -> (29.2112, -15.2095)
  line L39 (36.8198, -15.3653) -> (39.8452, -15.3653)
  line L40 (39.8452, -15.3653) -> (39.8452, -16.4961)
  line L41 (39.8452, -16.4961) -> (37.9707, -16.4961)
  line L42 (37.9707, -16.4961) -> (37.9707, -17.6017)
  line L43 (37.9707, -17.6017) -> (39.8452, -17.6017)
  line L44 (39.8452, -17.6017) -> (39.8452, -18.7174)
  line L45 (39.8452, -18.7174) -> (37.9707, -18.7174)
  line L46 (37.9707, -18.7174) -> (37.9707, -21.4613)
  line L47 (37.9707, -21.4613) -> (36.8198, -21.4613)
  line L48 (36.8198, -21.4613) -> (36.8198, -15.3653)
  line L49 (45.2678, -19.5315) -> (41.6394, -19.5315)
  spline S12 degree 2 poles (41.6394, -19.5315) (41.7198, -20.0139) (42.4032, -20.5818) (42.9309, -20.5818) knots 0 0 0 1 2 2 2
  spline S13 degree 2 poles (42.9309, -20.5818) (43.5641, -20.5818) (44.0215, -20.1396) knots 0 0 0 1 1 1
  line L50 (44.0215, -20.1396) -> (44.9713, -20.5869)
  spline S14 degree 2 poles (44.9713, -20.5869) (44.6145, -21.0894) (43.6194, -21.5769) (42.936, -21.5769) knots 0 0 0 1 2 2 2
  spline S15 degree 2 poles (42.936, -21.5769) (41.8756, -21.5769) (40.5438, -20.2401) (40.5438, -19.23) knots 0 0 0 1 2 2 2
  spline S16 degree 2 poles (40.5438, -19.23) (40.5438, -18.1997) (41.8756, -16.8378) (42.8756, -16.8378) knots 0 0 0 1 2 2 2
  spline S17 degree 2 poles (42.8756, -16.8378) (43.9411, -16.8378) (45.2728, -18.1997) (45.2728, -19.3154) knots 0 0 0 1 2 2 2
  line L51 (45.2728, -19.3154) -> (45.2678, -19.5315)
  spline S18 degree 2 poles (44.1371, -18.642) (44.0265, -18.2651) (43.3681, -17.7977) (42.9309, -17.7977) knots 0 0 0 1 2 2 2
  spline S19 degree 2 poles (42.9309, -17.7977) (42.4585, -17.7977) (42.1017, -18.059) knots 0 0 0 1 1 1
  spline S20 degree 2 poles (42.1017, -18.059) (41.8806, -18.2249) (41.6896, -18.642) knots 0 0 0 1 1 1
  line L52 (41.6896, -18.642) -> (44.1371, -18.642)
  line L53 (47.3132, -15.2095) -> (47.3132, -17.4509)
  spline S21 degree 2 poles (47.3132, -17.4509) (47.6198, -17.1444) (48.3334, -16.8378) (48.7354, -16.8378) knots 0 0 0 1 2 2 2
  spline S22 degree 2 poles (48.7354, -16.8378) (49.6199, -16.8378) (50.8512, -18.1696) (50.8512, -19.2149) knots 0 0 0 1 2 2 2
  spline S23 degree 2 poles (50.8512, -19.2149) (50.8512, -20.22) (49.5747, -21.5769) (48.7053, -21.5769) knots 0 0 0 1 2 2 2
  spline S24 degree 2 poles (48.7053, -21.5769) (48.3133, -21.5769) (47.6449, -21.3005) (47.3132, -20.9839) knots 0 0 0 1 2 2 2
  line L54 (47.3132, -20.9839) -> (47.3132, -21.4613)
  line L55 (47.3132, -21.4613) -> (46.1875, -21.4613)
  line L56 (46.1875, -21.4613) -> (46.1875, -15.2095)
  line L57 (46.1875, -15.2095) -> (47.3132, -15.2095)
  spline S25 degree 2 poles (48.4992, -17.8831) (47.9665, -17.8831) (47.263, -18.6118) (47.263, -19.1998) knots 0 0 0 1 2 2 2
  spline S26 degree 2 poles (47.263, -19.1998) (47.263, -19.7978) (47.9665, -20.5416) (48.4992, -20.5416) knots 0 0 0 1 2 2 2
  spline S27 degree 2 poles (48.4992, -20.5416) (49.0169, -20.5416) (49.7255, -19.7878) (49.7255, -19.2048) knots 0 0 0 1 2 2 2
  spline S28 degree 2 poles (49.7255, -19.2048) (49.7255, -18.6219) (49.032, -17.8831) (48.4992, -17.8831) knots 0 0 0 1 2 2 2
  line L58 (25.8692, -27.6921) -> (24.7384, -27.6921)
  spline S29 degree 2 poles (24.7384, -27.6921) (24.7836, -26.7071) (25.9345, -25.5764) (26.8341, -25.5764) knots 0 0 0 1 2 2 2
  spline S30 degree 2 poles (26.8341, -25.5764) (27.3869, -25.5764) (28.2412, -26.0437) (28.7488, -26.9282) (28.7488, -27.3805) knots 0 0 0 1 2 3 3 3
  spline S31 degree 2 poles (28.7488, -27.3805) (28.7488, -27.9233) (28.1307, -29.1747) (27.3065, -30.029) knots 0 0 0 1 2 2 2
  line L59 (27.3065, -30.029) -> (26.623, -30.7477)
  line L60 (26.623, -30.7477) -> (28.7991, -30.7477)
  line L61 (28.7991, -30.7477) -> (28.7991, -31.8231)
  line L62 (28.7991, -31.8231) -> (24.5726, -31.8231)
  line L63 (24.5726, -31.8231) -> (24.5726, -31.2703)
  line L64 (24.5726, -31.2703) -> (26.4622, -29.3455)
  spline S32 degree 2 poles (26.4622, -29.3455) (27.1457, -28.652) (27.598, -27.8127) (27.598, -27.476) knots 0 0 0 1 2 2 2
  spline S33 degree 2 poles (27.598, -27.476) (27.598, -27.1192) (27.1306, -26.6619) (26.7587, -26.6619) knots 0 0 0 1 2 2 2
  spline S34 degree 2 poles (26.7587, -26.6619) (26.3868, -26.6619) (25.8842, -27.2147) (25.8692, -27.6921) knots 0 0 0 1 2 2 2
  spline S35 degree 2 poles (31.5028, -25.5764) (32.1712, -25.5764) (33.1361, -26.2297) (33.6638, -27.5765) (33.6638, -28.7776) knots 0 0 0 1 2 3 3 3
  spline S36 degree 2 poles (33.6638, -28.7776) (33.6638, -29.9888) (33.1311, -31.3407) (32.2265, -31.9739) (31.538, -31.9739) knots 0 0 0 1 2 3 3 3
  spline S37 degree 2 poles (31.538, -31.9739) (30.8495, -31.9739) (29.9147, -31.3356) (29.382, -30.034) (29.382, -28.8329) knots 0 0 0 1 2 3 3 3
  spline S38 degree 2 poles (29.382, -28.8329) (29.382, -27.1594) (29.8997, -26.4056) knots 0 0 0 1 1 1
  spline S39 degree 2 poles (29.8997, -26.4056) (30.4776, -25.5764) (31.5028, -25.5764) knots 0 0 0 1 1 1
  spline S40 degree 2 poles (31.533, -26.677) (31.2365, -26.677) (30.7842, -27.0539) (30.5429, -27.9735) (30.5429, -28.858) knots 0 0 0 1 2 3 3 3
  spline S41 degree 2 poles (30.5429, -28.858) (30.5429, -30.0139) (31.0907, -30.8984) (31.533, -30.8984) knots 0 0 0 1 2 2 2
  spline S42 degree 2 poles (31.533, -30.8984) (31.9551, -30.8984) (32.2014, -30.4813) knots 0 0 0 1 1 1
  spline S43 degree 2 poles (32.2014, -30.4813) (32.5029, -29.9737) (32.5029, -28.7877) knots 0 0 0 1 1 1
  spline S44 degree 2 poles (32.5029, -28.7877) (32.5029, -27.5866) (31.9601, -26.677) (31.533, -26.677) knots 0 0 0 1 2 2 2
  line L65 (35.3775, -27.6921) -> (34.2468, -27.6921)
  spline S45 degree 2 poles (34.2468, -27.6921) (34.292, -26.7071) (35.4428, -25.5764) (36.3424, -25.5764) knots 0 0 0 1 2 2 2
  spline S46 degree 2 poles (36.3424, -25.5764) (36.8952, -25.5764) (37.7496, -26.0437) (38.2572, -26.9282) (38.2572, -27.3805) knots 0 0 0 1 2 3 3 3
  spline S47 degree 2 poles (38.2572, -27.3805) (38.2572, -27.9233) (37.639, -29.1747) (36.8148, -30.029) knots 0 0 0 1 2 2 2
  line L66 (36.8148, -30.029) -> (36.1313, -30.7477)
  line L67 (36.1313, -30.7477) -> (38.3074, -30.7477)
  line L68 (38.3074, -30.7477) -> (38.3074, -31.8231)
  line L69 (38.3074, -31.8231) -> (34.0809, -31.8231)
  line L70 (34.0809, -31.8231) -> (34.0809, -31.2703)
  line L71 (34.0809, -31.2703) -> (35.9705, -29.3455)
  spline S48 degree 2 poles (35.9705, -29.3455) (36.654, -28.652) (37.1063, -27.8127) (37.1063, -27.476) knots 0 0 0 1 2 2 2
  spline S49 degree 2 poles (37.1063, -27.476) (37.1063, -27.1192) (36.6389, -26.6619) (36.267, -26.6619) knots 0 0 0 1 2 2 2
  spline S50 degree 2 poles (36.267, -26.6619) (35.8951, -26.6619) (35.3926, -27.2147) (35.3775, -27.6921) knots 0 0 0 1 2 2 2
  line L72 (41.1117, -25.5764) -> (42.0967, -26.0689)
  line L73 (42.0967, -26.0689) -> (41.0363, -28.1444)
  spline S51 degree 2 poles (41.0363, -28.1444) (41.8102, -28.1444) (42.8957, -29.2551) (42.8957, -30.0742) knots 0 0 0 1 2 2 2
  spline S52 degree 2 poles (42.8957, -30.0742) (42.8957, -30.8683) (41.7801, -31.9739) (40.9961, -31.9739) knots 0 0 0 1 2 2 2
  spline S53 degree 2 poles (40.9961, -31.9739) (40.1669, -31.9739) (39.0713, -30.8281) (39.0713, -30.0893) knots 0 0 0 1 2 2 2
  spline S54 degree 2 poles (39.0713, -30.0893) (39.0713, -29.8079) (39.2422, -29.24) (39.5487, -28.647) knots 0 0 0 1 2 2 2
  line L74 (39.5487, -28.647) -> (41.1117, -25.5764)
  spline S55 degree 2 poles (40.971, -29.245) (40.6443, -29.245) (40.2071, -29.7124) (40.2071, -30.0592) knots 0 0 0 1 2 2 2
  spline S56 degree 2 poles (40.2071, -30.0592) (40.2071, -30.4109) (40.6644, -30.8884) (40.971, -30.8884) knots 0 0 0 1 2 2 2
  spline S57 degree 2 poles (40.971, -30.8884) (41.2976, -30.8884) (41.76, -30.421) (41.76, -30.0592) knots 0 0 0 1 2 2 2
  spline S58 degree 2 poles (41.76, -30.0592) (41.76, -29.7124) (41.3077, -29.245) (40.971, -29.245) knots 0 0 0 1 2 2 2
  point P0 (0, 0)
  point P1 (33.9, -39.75)
  point P2 (33.9, -38.6205)
  dimension "d0" = 79.5
  dimension "d42" = 129.1
  dimension "d29" = 0
  constraints: 2 midpoint, 2 other
  measures "d29" horizontal distance of point (33.9, -39.75) point (33.9, -38.62)
emboss "Emboss1" sketch "Sketch6" operation cut depth 1.5 direction (1, 0, 0)
emboss "Emboss2" sketch "Sketch7" operation cut depth 1.5 direction (1, 0, 0)
emboss "Emboss3" sketch "Sketch8" operation cut depth 1.5 direction (1, 0, 0)
fillet "Fillet1" radius 1 16 edges at (152.4, 0, 64.55) (0, 0, 64.55) (152.4, 0, -64.55) (0, 0, -64.55) (76.2, 39.75, -64.55) (152.4, 39.75, -33.9) (152.4, 39.75, 33.9) (76.2, 39.75, 64.55) (0, 39.75, 33.9) (0, 39.75, -33.9) (0, -39.75, -33.9) (0, -39.75, 33.9) (76.2, -39.75, 64.55) (152.4, -39.75, 33.9) (152.4, -39.75, -33.9) (76.2, -39.75, -64.55)
chamfer "Chamfer1" distance 3 distance2 6 1 edges at (77.3984, 39.75, -38.5) measured on face at (77.3984, 39.75, -39)
chamfer "Chamfer2" distance 3 distance2 6 1 edges at (77.3984, -39.75, -38.5) measured on face at (77.3984, -39.75, -39)
chamfer "Chamfer3" distance 3 distance2 6 1 edges at (77.3984, 39.75, 38.5) measured on face at (77.3984, 39.75, 39)
chamfer "Chamfer4" distance 3 distance2 6 1 edges at (77.3984, -39.75, 38.5) measured on face at (77.3984, -39.75, 39)
body "Solid1"
